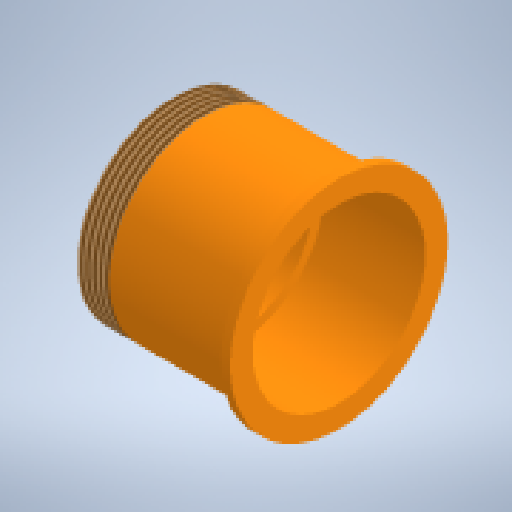
# Autodesk Inventor part: 030
Saved by Autodesk Inventor 2023 (Build 270158000, 158)
## iProperties
Created: 2022-04-04
Part Number: 030
Material: Aluminum 6061
Document SubType Name: Modeling
Designer: Vinicius Miguel
Density: 2.7 g/cm^3
Appearance: Orange
Mass: 5.38202 g
Surface Area: 28.7927 cm^2
Volume: 1.99334 cm^3
Author: Vinicius Miguel
Autodesk Inventor part; units mm, degrees
ref_plane "YZ Plane" through (0, 0, 0) normal (1, 0, 0) x (0, 1, 0)
ref_plane "XZ Plane" through (0, 0, 0) normal (0, 1, 0) x (-1, 0, 0)
ref_plane "XY Plane" through (0, 0, 0) normal (0, 0, 1) x (1, 0, 0)
sketch "Sketch1" plane through (0, 0, 0) normal (0, 1, 0) x (-1, 0, 0)
  line L0 (0, 0) -> (10, 0)
  line L1 (2, -13.5) -> (10, -13.5)
  line L2 (2, -13.5) -> (2, -12)
  line L3 (2, -12) -> (0, -12)
  line L4 (10, -15) -> (10, -13.5)
  line L5 (0, -13.5) -> (-16, -13.5)
  line L6 (0, -13.5) -> (0, -12)
  line L7 (-16, -13.5) -> (-16, -17)
  line L8 (-16, -17) -> (-14.5, -17)
  line L9 (-14.5, -17) -> (-14.5, -15)
  line L10 (10, -15) -> (-14.5, -15)
  dimension "d0" = 1.5
  dimension "d4" = 1.5
  dimension "d5" = 10
  dimension "d7" = 24
  dimension "d8" = 27
  dimension "d11" = 16
  dimension "d12" = 27
  dimension "d13" = 1.5
  dimension "d14" = 34
  dimension "d16" = 2
  constraints: 22 end point, 4 horizontal, 3 perpendicular, 3 vertical, 2 vertical alignment
  measures "d0" distance of L1.start L2.end
  measures "d4" distance of L4.start L1.end
  measures "d5" distance of L0.start L0.end
  measures "d7" diameter of L3 L0
  measures "d8" diameter of L1 L0
  measures "d11" distance of L5.start L5.end
  measures "d12" diameter of L5 L0
  measures "d13" distance of L7.end L8.end
  measures "d14" diameter of L7.end L0
  measures "d16" distance of L2.end L3.end
revolve "Revolution1" add sketch "Sketch1" angle 360 about axis through (0, 0, 0) along (-1, 0, 0)
thread "Thread1" size "M30x1" class "6g" standard "ANSI Metric M Profile" length 5
body "Solid1"
